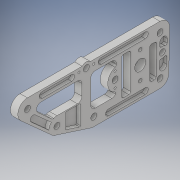
# Autodesk Inventor part: Frame_Bearing_New
Saved by Autodesk Inventor 2019 (Build 230136000, 136)
## iProperties
Created: 2019-10-21
Part Number: Frame_Bearing_New
Material: Generic
Document SubType Name: Modeling
Designer: 19879326
Density: 1 g/cm^3
Appearance: Default
Author: 19879326
Autodesk Inventor part; units mm, degrees
ref_plane "YZ Plane" through (0, 0, 0) normal (1, 0, 0) x (0, 1, 0)
ref_plane "XZ Plane" through (0, 0, 0) normal (0, 1, 0) x (-1, 0, 0)
ref_plane "XY Plane" through (0, 0, 0) normal (0, 0, 1) x (1, 0, 0)
sketch "Sketch1" plane through (0, 0, 0) normal (1, 0, 0) x (0, 1, 0)
  circle A0 centre (33, 0) radius 4
  circle A1 centre (-29, -10) radius 4
  circle A2 centre (-29, -100) radius 4
  circle A3 centre (25, 80) radius 4
  circle A4 centre (25, -100) radius 4
  arc A5 (38, -5.5902) -> (38, 5.5902) centre (33, 0) ccw
  line L0 (38, -5.5902) -> (38, -100)
  line L1 (38, 5.5902) -> (38, 80)
  arc A6 (38, 80) -> (15.333, 88.692) centre (25, 80) ccw
  arc A7 (24.7593, -112.9978) -> (38, -100) centre (25, -100) ccw
  circle A8 centre (0, -39) radius 4
  circle A9 centre (-15, 40) radius 4
  line L2 (-41, -10) -> (-41, -100)
  arc A10 (-41, -100) -> (-29.2222, -111.9979) centre (-29, -100) ccw
  arc A11 (-40.4224, -6.3217) -> (-41, -10) centre (-29, -10) ccw
  line L3 (24.7593, -112.9978) -> (-29.2222, -111.9979)
  arc A12 (-3, 40) -> (-4.4611, 45.7386) centre (-15, 40) ccw
  line L4 (-4.4611, 45.7386) -> (13.5383, 65.757)
  line L5 (24, 61.7453) -> (24, 12)
  line L6 (3, 6) -> (18, 6)
  arc A13 (24, 61.7453) -> (13.5383, 65.757) centre (18, 61.7453) ccw
  arc A14 (18, 6) -> (24, 12) centre (18, 12) ccw
  arc A15 (-3, 12) -> (3, 6) centre (3, 12) ccw
  line L7 (19.5175, -6) -> (-14, -6)
  arc A16 (24, -12) -> (18, -6) centre (18, -12) ccw
  arc A17 (18, -40.65) -> (24, -34.65) centre (18, -34.65) ccw
  arc A18 (-14, -6) -> (-20, -12) centre (-14, -12) ccw
  arc A19 (-20, -34.65) -> (-15, -40.5661) centre (-14, -34.65) ccw
  line L8 (24, -12) -> (24, -34.65)
  line L9 (-20, -34.65) -> (-20, -12)
  line L10 (18, -40.65) -> (15, -40.65)
  circle A20 centre (0, -73.15) radius 7.5
  circle A21 centre (18.25, -73.15) radius 2.5
  circle A22 centre (-18.25, -73.15) radius 2.5
  line L11 (24, -48) -> (-27, -48)
  line L12 (-27, -48) -> (-27, -60.15)
  line L13 (-27, -60.15) -> (24, -60.15)
  line L14 (24, -60.15) -> (24, -48)
  line L15 (17, -86.15) -> (-27, -86.15)
  line L16 (-27, -86.15) -> (-27, -94.6485)
  arc A23 (15, -40.65) -> (-15, -40.5661) centre (-0.0109, -44.4957) ccw
  circle A24 centre (0, -103.15) radius 4
  line L17 (-27, -94.6485) -> (17, -95.4635)
  line L18 (17, -86.15) -> (17, -95.4635)
  line L19 (15.333, 88.692) -> (-22.4361, 46.6861)
  line L20 (-24.5186, 43.0652) -> (-40.4224, -6.3217)
  arc A25 (-22.4361, 46.6861) -> (-24.5186, 43.0652) centre (-15, 40) ccw
  arc A26 (-3, 40) -> (-4.4611, 45.7386) centre (-15, 40) ccw
  line L21 (-3, 12) -> (-3, 40)
  point P0 (0, 0)
  point P1 (38, 41.5104)
  point P2 (38, -62.1387)
  point P3 (16.5, -40.65)
  point P4 (-17.5, -40.65)
  point P5 (0, -29)
  dimension "d0" = 8
  dimension "d1" = 8
  dimension "d2" = 8
  dimension "d3" = 8
  dimension "d4" = 80
  dimension "d5" = 100
  dimension "d6" = 62
  dimension "d7" = 90
  dimension "d8" = 10
  dimension "d9" = 15
  dimension "d10" = 5
  dimension "d13" = 8
  dimension "d14" = 39
  dimension "d25" = 8
  dimension "d27" = 12
  dimension "d28" = 24
  dimension "d29" = 24
  dimension "d30" = 24
  dimension "d31" = 33
  dimension "d34" = 14
  dimension "d35" = 6
  dimension "d37" = 6
  dimension "d38" = 6
  dimension "d42" = 6
  dimension "d46" = 9
  dimension "d47" = 14
  dimension "d70" = 1.65
  dimension "d71" = 18.25
  dimension "d72" = 18.25
  dimension "d73" = 15
  dimension "d74" = 5
  dimension "d75" = 5
  dimension "d76" = 34.15
  dimension "d77" = 13
  dimension "d78" = 13
  dimension "d80" = 14
  dimension "d81" = 14
  dimension "d82" = 9
  dimension "d84" = 14
  dimension "d119" = 15
  dimension "d120" = 10
  dimension "d123" = 15
  dimension "d128" = 8
  dimension "d129" = 30
  dimension "d140" = 8
  dimension "d150" = 8
  dimension "d154" = 40
  dimension "d155" = 15
  dimension "d156" = 14
  dimension "d158" = 10
  constraints: 44 end point, 33 point on circle, 27 centre point, 19 tangent, 9 vertical alignment, 7 coincident, 7 equal radius, 6 horizontal alignment, 6 parallel, 5 vertical, 4 horizontal, 3 perpendicular, 3 point on line, 1 midpoint
  measures "d0" diameter of A0
  measures "d1" horizontal distance of A0.centre A3.centre
  measures "d2" diameter of A3
  measures "d3" diameter of A4
  measures "d4" vertical distance of A0.centre A3.centre
  measures "d5" vertical distance of A4.centre A0.centre
  measures "d6" horizontal distance of A1.centre A0.centre
  measures "d7" distance of A2.centre A1.centre
  measures "d8" vertical distance of A1.centre A0.centre
  measures "d9" diameter of A5
  measures "d10" distance from line of L0 A0.centre
  measures "d13" diameter of A8
  measures "d14" distance of A8.centre point (0, 0)
  measures "d25" diameter of A9
  measures "d27" distance from line of L2 A1.centre
  measures "d28" diameter of A10
  measures "d29" diameter of A11
  measures "d30" diameter of A12
  measures "d31" distance of A0.centre point (0, 0)
  measures "d34" distance between parallel lines of L1 L5
  measures "d35" distance from line of point (0, 0) L6
  measures "d37" radius of A13
  measures "d38" distance from line of point (0, 0) L7
  measures "d42" radius of A16
  measures "d46" distance from line of A1.centre L9
  measures "d47" distance between parallel lines of L0 L8
  measures "d70" distance from line of L10 A8.centre
  measures "d71" distance of A20.centre A21.centre
  measures "d72" distance of A22.centre A20.centre
  measures "d73" diameter of A20
  measures "d74" diameter of A22
  measures "d75" diameter of A21
  measures "d76" distance of A8.centre A20.centre
  measures "d77" distance from line of L13 A20.centre
  measures "d78" distance from line of L15 A20.centre
  measures "d80" distance between parallel lines of L0 L14
  measures "d81" distance between parallel lines of L2 L12
  measures "d82" distance from line of L11 A8.centre
  measures "d84" distance between parallel lines of L2 L16
  measures "d119" horizontal distance of L10.end A8.centre
  measures "d120" distance of point (0, -29) A8.centre
  measures "d123" horizontal distance of A8.centre A19.end
  measures "d128" diameter of A24
  measures "d129" distance of A20.centre A24.centre
  measures "d140" distance from line of L17 A24.centre
  measures "d150" distance from line of L18 A7.centre
  measures "d154" vertical distance of point (0, 0) A9.centre
  measures "d155" horizontal distance of point (0, 0) A9.centre
  measures "d156" distance between parallel lines of L19 L4
  measures "d158" radius of A25
extrude "Extrusion1" add sketch "Sketch1" along normal blind 10
fillet "Fillet1" radius 2.5 8 edges at (5, 24, -60.15) (5, 24, -48) (5, -27, -48) (5, -27, -60.15) (5, 17, -95.4635) (5, 17, -86.15) (5, -27, -94.6485) (5, -27, -86.15)
fillet "Fillet2" radius 2.5 3 edges at (5, 15, -40.65) (5, -4.4611, 45.7386) (5, -3, 40)
sketch "Sketch4" plane through (10, 0, 0) normal (1, 0, 0) x (0, 0, -1)
  arc A0 (-60, 35.5) -> (-60, 27.5) centre (-60, 31.5) ccw
  arc A1 (-20, 27.5) -> (-20, 35.5) centre (-20, 31.5) ccw
  arc A2 (20, 35.5) -> (20, 27.5) centre (20, 31.5) ccw
  arc A3 (80, 27.5) -> (80, 35.5) centre (80, 31.5) ccw
  line L0 (-60, 35.5) -> (-20, 35.5)
  line L1 (-60, 27.5) -> (-20, 27.5)
  line L2 (20, 35.5) -> (80, 35.5)
  line L3 (20, 27.5) -> (80, 27.5)
  line L4 (-5.5902, 38) -> (-80, 38) projected
  circle A4 centre (-80, 25) radius 4 projected
  circle A5 centre (0, 33) radius 4 projected
  circle A6 centre (100, 25) radius 4 projected
  arc A7 (-69.6168, 12.9744) -> (-74.9657, 7.0256) centre (-72.2912, 10) ccw
  arc A8 (30, -30) -> (30, -38) centre (30, -34) ccw
  arc A9 (80, -38) -> (80, -30) centre (80, -34) ccw
  line L5 (30, -38) -> (80, -38)
  line L6 (30, -30) -> (80, -30)
  line L7 (10, -41) -> (100, -41) projected
  circle A10 centre (10, -29) radius 4 projected
  circle A11 centre (-40, -15) radius 4 projected
  line L8 (-69.6168, 12.9744) -> (-47.4772, -6.9321)
  circle A12 centre (100, -29) radius 4 projected
  arc A13 (109.7777, 12.9074) -> (99.7795, 13.0926) centre (104.7786, 13) ccw
  arc A14 (99.2238, -16.9074) -> (109.2221, -17.0926) centre (104.2229, -17) ccw
  line L9 (97.5032, 19.4537) -> (97.3, 8.4853) projected
  line L10 (111.9979, -29.2222) -> (112.9978, 24.7593) projected
  circle A15 centre (103.15, 0) radius 4 projected
  circle A16 centre (-40, -15) radius 4 projected
  line L11 (99.2238, -16.9074) -> (99.4272, -5.9279)
  line L12 (99.6492, 6.0617) -> (99.7795, 13.0926)
  arc A17 (109.7777, 12.9074) -> (99.7795, 13.0926) centre (104.7786, 13) ccw
  arc A18 (99.2238, -16.9074) -> (109.2221, -17.0926) centre (104.2229, -17) ccw
  line L13 (99.2238, -16.9074) -> (99.4272, -5.9279)
  line L14 (99.7795, 13.0926) -> (99.6492, 6.0617)
  arc A19 (99.4272, -5.9279) -> (109.4835, -2.9812) centre (103.15, 0) ccw
  arc A20 (109.5895, 2.7446) -> (99.6492, 6.0617) centre (103.15, 0) ccw
  line L15 (109.7777, 12.9074) -> (109.5895, 2.7446)
  line L16 (109.4835, -2.9812) -> (109.2221, -17.0926)
  arc A21 (99.4272, -5.9279) -> (109.4835, -2.9812) centre (103.15, 0) ccw
  arc A22 (109.5895, 2.7446) -> (99.6492, 6.0617) centre (103.15, 0) ccw
  line L17 (109.7777, 12.9074) -> (109.5895, 2.7446)
  line L18 (109.4835, -2.9812) -> (109.2221, -17.0926)
  line L19 (109.2221, -17.0926) -> (109.4835, -2.9812)
  line L20 (109.5895, 2.7446) -> (109.7777, 12.9074)
  line L21 (-74.9657, 7.0256) -> (-50.99, -14.5319)
  arc A23 (-47.4772, -6.9321) -> (-50.99, -14.5319) centre (-40, -15) ccw
  line L22 (-46.9639, -3.3594) -> (-65.757, 13.5383) projected
  line L23 (-88.692, 15.333) -> (-46.6861, -22.4361) projected
  line L24 (-28, -4.5) -> (-8, -4.5)
  line L25 (-8, -4.5) -> (-8, -31.9405)
  line L26 (-28, -25.5) -> (-28, -4.5)
  line L27 (-28, -25.5) -> (-8, -31.9405)
  line L28 (-43.0652, -24.5186) -> (6.3217, -40.4224) projected
  point P0 (0, 0)
  point P1 (98.2303, -9.5463)
  point P2 (97.3, 8.4853)
  point P3 (-28, -15)
  dimension "d88" = 8
  dimension "d89" = 2.5
  dimension "d90" = 20
  dimension "d91" = 20
  dimension "d92" = 20
  dimension "d93" = 20
  dimension "d96" = 8
  dimension "d97" = 15
  dimension "d101" = 20
  dimension "d102" = 20
  dimension "d103" = 3
  dimension "d104" = 10
  dimension "d106" = 12
  dimension "d107" = 12
  dimension "d146" = 3
  dimension "d147" = 7
  dimension "d148" = 7
  dimension "d152" = 11
  dimension "d159" = 3
  dimension "d162" = 21
  dimension "d163" = 12
  dimension "d164" = 20
  constraints: 44 end point, 32 point on circle, 16 centre point, 15 tangent, 14 parallel, 6 equal radius, 5 point on line, 4 coincident, 2 horizontal, 1 collinear, 1 horizontal alignment, 1 midpoint, 1 perpendicular, 1 other
  measures "d88" diameter of A0
  measures "d89" distance between parallel lines of L4 L0
  measures "d90" horizontal distance of A4.centre A0.centre
  measures "d91" horizontal distance of A1.centre A5.centre
  measures "d92" horizontal distance of A2.centre A5.centre
  measures "d93" horizontal distance of A6.centre A3.centre
  measures "d96" diameter of A7
  measures "d97" vertical distance of A7.centre A4.centre
  measures "d101" horizontal distance of A8.centre A10.centre
  measures "d102" horizontal distance of A12.centre A9.centre
  measures "d103" distance between parallel lines of L7 L5
  measures "d104" diameter of A13
  measures "d106" vertical distance of A13.centre A6.centre
  measures "d107" vertical distance of A12.centre A14.centre
  measures "d146" distance between parallel lines of L10 L15
  measures "d147" radius of A20
  measures "d148" radius of A19
  measures "d152" radius of A23
  measures "d159" distance between parallel lines of L23 L21
  measures "d162" distance of L26.start L24.start
  measures "d163" distance from line of L26 A11.centre
  measures "d164" distance of L24.start L24.end
extrude "Extrusion3" cut sketch "Sketch4" against normal blind 5 contours L0 A1 L1 A0 | L2 A3 L3 A2 | L8 A23 L21 A7 | L6 A9 L5 A8 | L15 A20 L12 A13 | L11 A19 L16 A14 | L24 L25 L27 L26
sketch "Sketch5" plane through (10, 0, 0) normal (1, 0, 0) x (0, 0, -1)
  circle A0 centre (39, -10) radius 1.5
  circle A1 centre (39, 10) radius 1.5
  circle A2 centre (39, 0) radius 4 projected
  circle A3 centre (-10, 33) radius 1.5
  circle A4 centre (10, 33) radius 1.5
  circle A5 centre (0, 33) radius 4 projected
  circle A6 centre (103.15, 10) radius 1.5
  circle A7 centre (103.15, -10) radius 1.5
  circle A8 centre (103.15, 0) radius 4 projected
  point P0 (0, 0)
  dimension "d109" = 3
  dimension "d110" = 3
  dimension "d113" = 3
  dimension "d114" = 3
  dimension "d115" = 10
  dimension "d116" = 10
  dimension "d117" = 10
  dimension "d118" = 10
  dimension "d136" = 3
  dimension "d137" = 3
  dimension "d138" = 10
  dimension "d139" = 10
  constraints: 6 centre point, 4 vertical alignment, 2 horizontal alignment
  measures "d109" diameter of A0
  measures "d110" diameter of A1
  measures "d113" diameter of A3
  measures "d114" diameter of A4
  measures "d115" distance of A5.centre A3.centre
  measures "d116" distance of A4.centre A5.centre
  measures "d117" distance of A2.centre A1.centre
  measures "d118" distance of A0.centre A2.centre
  measures "d136" diameter of A6
  measures "d137" diameter of A7
  measures "d138" distance of A8.centre A6.centre
  measures "d139" distance of A8.centre A7.centre
extrude "Extrusion4" cut sketch "Sketch5" against normal blind 10 contours A0 | A1 | A3 | A4 | A6 | A7
fillet "Fillet3" radius 2 1 edges at (5, -15, -40.5661)
fillet "Fillet6" radius 2 2 edges at (7.5, 6.0617, -99.6492) (7.5, -5.9279, -99.4272)
fillet "Fillet7" radius 2 2 edges at (7.5, 2.7446, -109.5895) (7.5, -2.9812, -109.4835)
fillet "Fillet9" radius 1 4 edges at (7.5, -31.9405, 8) (7.5, -25.5, 28) (7.5, -4.5, 28) (7.5, -4.5, 8)
body "Solid1"
